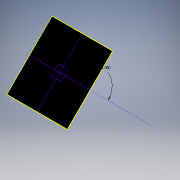
# Autodesk Inventor part: BackV1
Saved by Autodesk Inventor 2019 (Build 230136000, 136)
## iProperties
Created: 2021-09-16
Part Number: BackV1
Material: Aluminum 6061
Document SubType Name: Modeling
Designer: timmy
Density: 2.7 g/cm^3
Appearance: Aluminum - Flat
Author: timmy
Autodesk Inventor part; units mm, degrees
ref_plane "YZ Plane" through (0, 0, 0) normal (1, 0, 0) x (0, 1, 0)
ref_plane "XZ Plane" through (0, 0, 0) normal (0, 1, 0) x (-1, 0, 0)
ref_plane "XY Plane" through (0, 0, 0) normal (0, 0, 1) x (1, 0, 0)
sketch "Sketch6" plane through (0, 0, 0) normal (0, 1, 0) x (-1, 0, 0)
  line L0 (0, 0) -> (609.6, 0)
  line L1 (609.6, 0) -> (609.6, -914.4)
  line L2 (609.6, -914.4) -> (0, -914.4)
  line L3 (0, -914.4) -> (0, 0)
  dimension "d21" = 609.6
  dimension "d22" = 914.4
  constraints: 8 end point, 2 parallel, 1 horizontal, 1 perpendicular
  measures "d21" distance of L1.end L2.end
  measures "d22" distance of L0.end L1.end
extrude "Extrusion6" add sketch "Sketch6" along normal blind 609.6
sketch "Sketch8" plane through (0, 0, 0) normal (1, 0, 0) x (0, 0, -1)
  line L0 (0, 609.6) -> (914.4, 609.6) projected
  line L1 (0, 0) -> (457.2, 0) construction
  line L2 (0, 0) -> (457.2, 457.2)
  line L3 (0, 0) -> (646.5784, 0) construction
  line L4 (457.2, 457.2) -> (914.4, 0)
  line L5 (457.2, 457.2) -> (459.4451, 454.9549)
  line L6 (0, 0) -> (3.175, 0)
  line L7 (3.175, 0) -> (459.4451, 454.9549)
  dimension "d29" = 45
  dimension "d30" = 3.175
  dimension "d31" = 3.175
  constraints: 14 end point, 2 horizontal, 2 point on line, 1 equal length, 1 perpendicular
  measures "d29" angle of L3 L2
  measures "d30" distance of L2.end L5.end
  measures "d31" distance of L1.start L6.end
extrude "Extrusion7" cut sketch "Sketch8" against normal blind 609.6 keep common part
sketch "Sketch9" plane through (-609.6, 457.2, -457.2) normal (0, 0.7071068, 0.7071068) x (1, 0, 0)
  line L0 (609.6, -646.5784) -> (609.6, 0) projected
  line L1 (609.6, 0) -> (0, 0) projected
  line L2 (0, 0) -> (0, -646.5784) projected
  line L3 (609.6, -646.5784) -> (0, -646.5784) projected
  line L4 (609.6, -646.5784) -> (0, -646.5784) projected
  line L5 (304.8, -646.5784) -> (304.8, 0)
  line L6 (609.6, 0) -> (0, 0) projected
  line L7 (609.6, -646.5784) -> (609.6, 0) projected
  line L8 (609.6, -323.2892) -> (0, -323.2892)
  line L9 (0, 0) -> (0, -646.5784) projected
  line L10 (609.6, -323.2892) -> (1219.2, -323.2892) construction
  line L11 (355.6, -374.0892) -> (254, -374.0892)
  line L12 (254, -374.0892) -> (254, -272.4892)
  line L13 (254, -272.4892) -> (355.6, -272.4892)
  line L14 (355.6, -272.4892) -> (355.6, -374.0892)
  line L15 (355.6, -374.0892) -> (254, -272.4892) construction
  line L16 (254, -374.0892) -> (355.6, -272.4892) construction
  point P0 (304.8, -323.2892)
  dimension "d34" = 180
  dimension "d35" = 101.6
  dimension "d36" = 101.6
  constraints: 18 end point, 7 midpoint, 2 horizontal, 2 parallel, 1 collinear, 1 perpendicular
  measures "d34" angle of L8 L10
  measures "d35" distance of L12.end L13.end
  measures "d36" distance of L11.end L12.end
body "Solid4"
